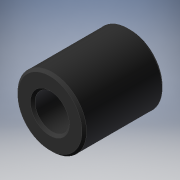
# Autodesk Inventor part: FWSSA-D6-V3-T7
Saved by Autodesk Inventor 2019 (Build 230136000, 136)
## iProperties
Created: 2022-12-28
Part Number: FWSSA-D6-V3-T7
Material: Generic
Catalog Web Link: www.cadenas.de
Description: FWS, FWSSC, FWSSB, FWSSM, FWSSR, FWSA,FWSSA, FWSSAB, FWSBB, FWSSS, FWSSSR, FWSUS-Metal Washers - Standard Grade - Dimension Configurable -
Vendor: MISUMI
Document SubType Name: Modeling
Designer: psAdmin
Manufacturer: MISUMI
Mass: 0.147309 g
Surface Area: 2.33707 cm^2
Volume: 0.147309 cm^3
Density: 1 g/cm^3
Appearance: PSOLRGB-175-175-175
Category: PARTsolutions
Company: MISUMI
Title: FWSSA-D6-V3-T7
Author: Cadenas PARTsolutions
Comments: Metal Washers - Standard Grade - Dimension Configurable -
PSOL_IDENT_0: {$CADENAS_DATA/23d-libs/misumi/metric/26_washers_collars/fwssc.prj},336 {VTYP=3D},{NB=FWSSA-D6-V3-T7
PSOL_IDENT_1: },{LINA=FWSSA-D6-V3-T7},{NN=FWS, FWSSC, FWSSB, FWSSM, FWSSR, FWSA,FWSSA, FWSSAB, FWSBB, FWSSS, FWSSS
PSOL_IDENT_2: R, FWSUS},{DATE=07.06.2021 03:25:40},{GEOMDATE=21.11.2019 05:40:01},{VERSION=},{LINEID=10},{WBVAR=MA
PSOL_IDENT_3: T,ST,D,ALT7,V,T,ALT1,ALT2,SC,WSC,ALT3,ALT4,ALT8,CC,WCC,ALT9,CV,WCV},{WBNUMERIC=D,V,T,SC,WSC,CC,WCC,C
PSOL_IDENT_4: V,WCV}  {NB=FWSSA-D6-V3-T7},{LINA=FWSSA-D6-V3-T7},{KT=DUMMY},{PN=FWSSA-D6-V3-T7},{TYPE=FWSSA},{TP=FW
PSOL_IDENT_5: S, FWSSC, FWSSB, FWSSM, FWSSR, FWSA,FWSSA, FWSSAB, FWSBB, FWSSS, FWSSSR, FWSUS},{MAT=2},{MATALG='7','
PSOL_IDENT_6: Low Carbon Steel','1' , '1045 Carbon Steel' ,'2' , 'Aluminum Alloy 2000 series' , '3' , 'Brass(C3604
PSOL_IDENT_7: )' , '4' , 'SUS304' ,'5' ,'SUS316(316 Stainless Steel)(1.4401_X5CrNiMo17-12-2)'},{ST=A},{STALG='-','
PSOL_IDENT_8: -','A','Alumite (Clear)','AB','Alumite (Black)'},{D=6.0},{DALG=[4:20/0.5],[21:100/1]},{ALT7=},{ALT7A
PSOL_IDENT_9: LG= '','w/o WVE (I.D. Dimension)','WVE','with WVE (I.D. Dimension)' },{V=3.0},{VMAX=0,2,2.6,[3:4/0.5
PSOL_IDENT_10: ]},{VI=0,2,2.6},{ALT7PN=-V3},{T=7.0},{TALG=[2:10/0.1]},{C=0.2},{D2=4.0},{D4=2.0},{D6=0},{D8=-2},{D10=
PSOL_IDENT_11: -4},{ALT1=},{ALT1AA=},{BB=0},{TT=0.0},{ALT1ALG='','Not applicable'},{ALT2=},{ALT2ALG='','Not applica
PSOL_IDENT_12: ble'},{SCMIN=4},{SCMAX=2},{SCALG=0},{SC=0},{ALT2AA=},{WSC=0},{WSCALG=0},{WSCMIN=7},{WSCMAX=5},{ALT3=
PSOL_IDENT_13: },{ALT4A='','w/o VKC (Inner Diameter Tolerance)','W','with VKC (Inner Diameter Tolerance)'},{ALT4TYP
PSOL_IDENT_14: E=T},{DV=T},{DV1=T},{ALT4AA=},{ALT4=},{ALT5A='','w/o Outer Diameter Tolerances','DKC','with DKC (Out
PSOL_IDENT_15: er Diameter Tolerance (g6))','HKC','with HKC (Outer Diameter Tolerance (h7))'},{ALT5AA=},{ALT8=},{AL
PSOL_IDENT_16: T8ALG= '','w/o O.D. C Chamfering','CC','with CC (O.D. C Chamfering (One Side))','WCC','with WCC (O.D
PSOL_IDENT_17: . C Chamfering (Both Side))' },{ALT8PN=},{CC=0},{CCALG=[0]},{CCMAX=0.5},{CCMAX1=1.5},{CCMAXALG=0.5},
PSOL_IDENT_18: {WCC=0},{WCCALG=[0]},{WCCMAX=0.5},{IDC=0.2},{ALT9=},{ALT9ALG= '','w/o I.D. C Chamfering','CV','with
PSOL_IDENT_19: CV (I.D. C Chamfering (One Side))','WCV','with WCV (I.D. C Chamfering (Both Sides))' },{ALT9PN=},{CV=
PSOL_IDENT_20: 0},{CVALG=[0]},{CVMAX=0.5},{CVMAX1=1.5},{CVMAXALG=0.5},{WCV=0},{WCVALG=[0]},{WCVMAX=0.5}
NB: FWSSA-D6-V3-T7
NN: FWS, FWSSC, FWSSB, FWSSM, FWSSR, FWSA,FWSSA, FWSSAB, FWSBB, FWSSS, FWSSSR, FWSUS
NT: Metal Washers - Standard Grade - Dimension Configurable -
NBSYN: $PN.
LINA: FWSSA-D6-V3-T7
CATALOG: Misumi
PN: FWSSA-D6-V3-T7
TP: FWS, FWSSC, FWSSB, FWSSM, FWSSR, FWSA,FWSSA, FWSSAB, FWSBB, FWSSS, FWSSSR, FWSUS
MAT: Aluminum Alloy 2000 series
ST: Alumite (Clear)
D: 6
ALT7: w/o WVE (I.D. Dimension)
V: 3
T: 7
ALT1: Not applicable
ALT2: Not applicable
SC: 0
WSC: 0
ALT3: w/o VKC (Inner Diameter Tolerance)
ALT4: w/o Outer Diameter Tolerances
ALT8: w/o O.D. C Chamfering
CC: 0
WCC: 0
ALT9: w/o I.D. C Chamfering
CV: 0
WCV: 0
SUPPLIER: MISUMI
ARTICLENO: FWSSA-D6-V3-T7
BOMINFO: FWSSA-D6-V3-T7
CREATOR: CADENAS GmbH
Autodesk Inventor part; units mm, degrees
sketch "_____1" plane through (0, 0, 0) normal (0, 1, 0) x (1, 0, 0)
  line L0 (0, 0) -> (0, 7)
  line L1 (0, 7) -> (3, 7)
  line L2 (3, 7) -> (3, 0)
  line L3 (3, 0) -> (0, 0)
  line L4 (0, 0) -> (0, 7)
  constraints: 10 end point
revolve "Revolution1" add sketch "_____1" angle 360 about axis through (0, 0, 0) along (0, 0, 1)
sketch "_____2" plane through (0, 0, 0) normal (0, 1, 0) x (1, 0, 0)
  line L0 (0, 0) -> (0, 7)
  line L1 (2.8, 7) -> (3, 6.8)
  line L2 (3, 6.8) -> (3, 7)
  line L3 (3, 7) -> (2.8, 7)
  constraints: 8 end point
revolve "Revolution2" cut sketch "_____2" angle 360 about axis through (0, 0, 0) along (0, 0, 1)
sketch "_____3" plane through (0, 0, 0) normal (0, 1, 0) x (1, 0, 0)
  line L0 (0, 0) -> (0, 7)
  line L1 (2.8, 0) -> (3, 0)
  line L2 (3, 0) -> (3, 0.2)
  line L3 (3, 0.2) -> (2.8, 0)
  constraints: 8 end point
revolve "Revolution3" cut sketch "_____3" angle 360 about axis through (0, 0, 0) along (0, 0, 1)
sketch "Sketch4" plane through (0, 0, 0) normal (0, 0, 1) x (1, 0, 0)
  point P0 (0, 0)
hole "Hole1" at (0, 0, 0) direction (0, 0, -1) diameter 3 depth 7
sketch "_____5" plane through (0, 0, 0) normal (0, 1, 0) x (1, 0, 0)
  line L0 (0, -14) -> (0, 14)
  line L1 (1.5, 6.8) -> (1.7, 7)
  line L2 (1.7, 7) -> (1.5, 7)
  line L3 (1.5, 7) -> (1.5, 6.8)
  constraints: 8 end point
revolve "Revolution4" cut sketch "_____5" angle 360 about axis through (0, 0, 14) along (0, 0, 1)
sketch "_____6" plane through (0, 0, 0) normal (0, 1, 0) x (1, 0, 0)
  line L0 (0, -14) -> (0, 14)
  line L1 (1.5, 0.2) -> (1.5, 0)
  line L2 (1.5, 0) -> (1.7, 0)
  line L3 (1.7, 0) -> (1.5, 0.2)
  constraints: 8 end point
revolve "Revolution5" cut sketch "_____6" angle 360 about axis through (0, 0, 14) along (0, 0, 1)
ref_plane "spring_XY" through (0, 0, 0) normal (0, 0, 1) x (1, 0, 0)
ref_plane "spring_YZ" through (0, 0, 0) normal (1, 0, 0) x (0, 1, 0)
ref_plane "spring_ZX" through (0, 0, 0) normal (0, 1, 0) x (0, 0, 1)
ref_plane "to_bolt_XY" through (0, 0, -7) normal (0, 0, 1) x (1, 0, 0)
ref_plane "to_bolt_YZ" through (0, 0, -7) normal (1, 0, 0) x (0, 1, 0)
ref_plane "to_bolt_ZX" through (0, 0, -7) normal (0, 1, 0) x (0, 0, 1)
body "Solid1"
